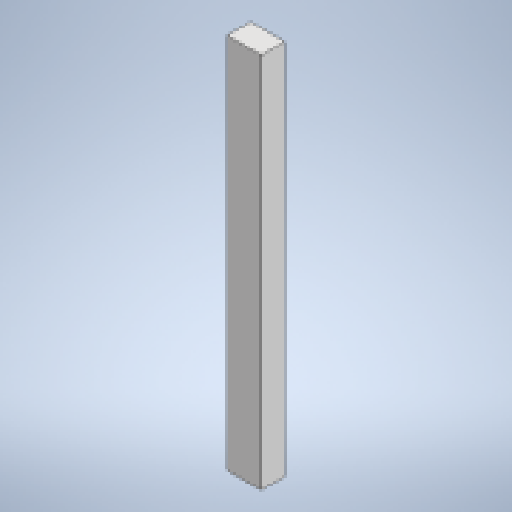
# Autodesk Inventor part: Нога для постели №2
Saved by Autodesk Inventor 2025 (Build 290162010, 162A)
## iProperties
Created: 2025-08-21
Part Number: Нога для постели №2
Material: Generic
Document SubType Name: Modeling
Designer: pokla
Density: 1 g/cm^3
Appearance: Default
Author: pokla
Autodesk Inventor part; units mm, degrees
ref_plane "YZ Plane" through (0, 0, 0) normal (1, 0, 0) x (0, 1, 0)
ref_plane "XZ Plane" through (0, 0, 0) normal (0, 1, 0) x (-1, 0, 0)
ref_plane "XY Plane" through (0, 0, 0) normal (0, 0, 1) x (1, 0, 0)
sketch "Sketch1" plane through (0, 0, 0) normal (0, 0, 1) x (1, 0, 0)
  line L0 (-32.813, 22.5) -> (32.813, 22.5)
  line L1 (32.813, 22.5) -> (32.813, -22.5)
  line L2 (32.813, -22.5) -> (-32.813, -22.5)
  line L3 (-32.813, -22.5) -> (-32.813, 22.5)
  line L4 (-32.813, 22.5) -> (32.813, -22.5) construction
  point P0 (0, 0)
  point P1 (0, 0)
  dimension "d0" = 65.626
  dimension "d1" = 45
  constraints: 10 end point, 2 parallel, 1 coincident, 1 horizontal, 1 midpoint, 1 perpendicular
  measures "d0" distance of L1.end L2.end
  measures "d1" distance of L2.end L0.start
extrude "Extrusion1" add sketch "Sketch1" along normal blind 725
body "Solid1"
